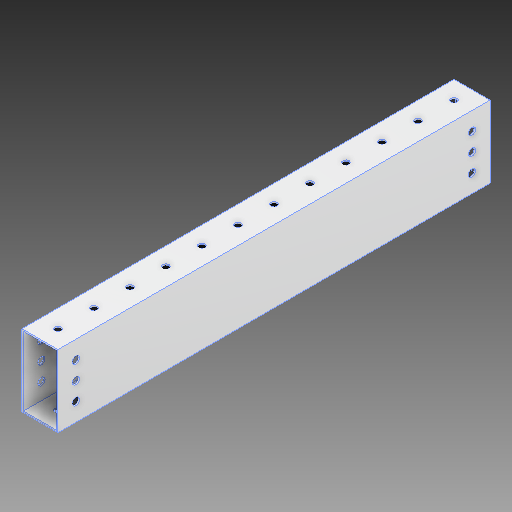
# Autodesk Inventor part: Elevator Stage 1 Gearbox Mounting Tube
Saved by Autodesk Inventor 2022 (Build 260153000, 153)
## iProperties
Created: 2020-09-06
Part Number: Elevator Stage 1 Gearbox Mounting Tube
Material: Aluminum 6061
Document SubType Name: Modeling
Density: 2.7 g/cm^3
Appearance: Aluminum - Flat
Autodesk Inventor part; units mm, degrees
ref_plane "YZ Plane" through (0, 0, 0) normal (1, 0, 0) x (0, 1, 0)
ref_plane "XZ Plane" through (0, 0, 0) normal (0, 1, 0) x (-1, 0, 0)
ref_plane "XY Plane" through (0, 0, 0) normal (0, 0, 1) x (1, 0, 0)
sketch "Sketch1" plane through (0, 0, 0) normal (0, 0, 1) x (1, 0, 0)
  line L0 (12.7, 25.4) -> (-12.7, 25.4)
  line L1 (-12.7, 25.4) -> (-12.7, -25.4)
  line L2 (-12.7, -25.4) -> (12.7, -25.4)
  line L3 (12.7, -25.4) -> (12.7, 25.4)
  line L4 (12.7, 25.4) -> (-12.7, -25.4) construction
  line L5 (-12.7, 25.4) -> (12.7, -25.4) construction
  line L6 (-11.684, 24.384) -> (11.684, 24.384)
  line L7 (11.684, 24.384) -> (11.684, -24.384)
  line L8 (11.684, -24.384) -> (-11.684, -24.384)
  line L9 (-11.684, -24.384) -> (-11.684, 24.384)
  point P0 (0, 0)
  dimension "d0" = 1.016
  dimension "d1" = 50.8
  dimension "d2" = 25.4
  constraints: 20 end point, 4 parallel, 2 midpoint, 2 perpendicular, 1 horizontal, 3 other
  measures "d0" distance between parallel lines of L0 L6
  measures "d1" distance between parallel lines of L2 L0
  measures "d2" distance between parallel lines of L1 L3
extrude "Tube Length" add sketch "Sketch1" along normal mid plane 304.8
sketch "Sketch2" plane through (-12.7, 25.4, 152.4) normal (0, 1, 0) x (1, 0, 0)
  line L0 (0, 0) -> (0, 304.8) projected
  line L1 (25.4, 0) -> (0, 0) projected
  line L2 (25.4, 304.8) -> (25.4, 0) projected
  line L3 (0, 304.8) -> (25.4, 304.8) projected
  line L4 (25.4, 0) -> (0, 0) projected
  line L5 (12.7, 0) -> (12.7, 12.7) construction
  circle A0 centre (12.7, 12.7) radius 2.2479
  point P0 (12.7, 152.4)
  dimension "d5" = 12.7
  dimension "d6" = 4.4958
  constraints: 2 end point, 1 centre point, 1 coincident, 1 midpoint, 1 vertical
  measures "d5" distance of L5.start L5.end
  measures "d6" diameter of A0
extrude "Top Hole" cut sketch "Sketch2" against normal through all contours A0
pattern_linear "Rectangular Pattern1" count 12 spacing 25.4 along (0, 0, -1) of "Top Hole"
sketch "Sketch4" plane through (-12.7, -25.4, 152.4) normal (-1, 0, 0) x (0, 0, 1)
  line L0 (-304.8, 0) -> (0, 0) projected
  line L1 (0, 50.8) -> (0, 0) projected
  line L2 (0, 50.8) -> (-304.8, 50.8) projected
  line L3 (-304.8, 0) -> (-304.8, 50.8) projected
  line L4 (-304.8, 25.4) -> (-292.1, 25.4)
  line L5 (-152.4, 25.4) -> (-152.4, 13.4487)
  point P0 (-292.1, 12.7)
  point P1 (-292.1, 38.1)
  point P2 (-12.7, 12.7)
  point P3 (-12.7, 25.4)
  point P4 (-12.7, 38.1)
  dimension "d31" = 12.7
  dimension "d34" = 12.7
  constraints: 4 end point, 3 symmetric about line, 2 vertical, 1 coincident, 1 horizontal, 1 midpoint, 2 other
  measures "d31" distance of L4.start L4.end
  measures "d34" distance of point (-292.1, 12.7) point (-292.1, 25.4)
hole "Hole1" at (-12.7, -12.7, -139.7) at (-12.7, 0, -139.7) at (-12.7, 12.7, -139.7) at (-12.7, 12.7, 139.7) at (-12.7, -12.7, 139.7) at (-12.7, 0, 139.7) direction (1, 0, 0) diameter 5.1054 end through all clearance for "Flat Head Machine Screw (82)" size "#10" standard "Ansi Unified Screw Threads"
sketch "Sketch3" plane through (0, 0, 152.4) normal (0, 0, 1) x (1, 0, 0)
  line L0 (0, 0) -> (0, 25.4) construction
  line L1 (12.7, 25.4) -> (-12.7, 25.4) projected
  line L2 (-0.0508, 25.4) -> (0, 25.2984)
  line L3 (0.0508, 25.4) -> (0, 25.2984)
  line L4 (-12.7, 12.6492) -> (-12.5984, 12.7)
  line L5 (-12.7, 12.7508) -> (-12.5984, 12.7)
  line L6 (-12.7, -0.0508) -> (-12.5984, 0)
  line L7 (-12.7, 0.0508) -> (-12.5984, 0)
  line L8 (-12.7, -12.7508) -> (-12.5984, -12.7)
  line L9 (-12.7, -12.6492) -> (-12.5984, -12.7)
  line L10 (12.7, 0.0508) -> (12.5984, 0)
  line L11 (12.7, 12.6492) -> (12.5984, 12.7)
  line L12 (12.7, 12.7508) -> (12.5984, 12.7)
  line L13 (12.7, -0.0508) -> (12.5984, 0)
  line L14 (12.7, -12.6492) -> (12.5984, -12.7)
  line L15 (12.7, -12.7508) -> (12.5984, -12.7)
  line L16 (0.0508, -25.4) -> (0, -25.2984)
  line L17 (-0.0508, -25.4) -> (0, -25.2984)
  line L18 (-12.7, 25.4) -> (-12.7, -25.4) projected
  line L19 (12.7, -25.4) -> (12.7, 25.4) projected
  line L20 (-12.7, -25.4) -> (12.7, -25.4) projected
  point P0 (0, 12.7)
  point P1 (-12.7, 12.7)
  point P2 (-12.7, 0)
  point P3 (-12.7, -12.7)
  point P4 (12.7, 12.7)
  point P5 (12.7, 0)
  point P6 (12.7, -12.7)
  point P7 (0, -25.4)
  dimension "d12" = 0.1016
  dimension "d13" = 0.1016
  dimension "d16" = 90
  dimension "d20" = 12.7
  dimension "d27" = 360
  constraints: 34 end point, 3 point on line, 2 midpoint, 2 vertical, 1 equal length, 70 other
  measures "d12" distance of L3.start L2.start
  measures "d13" distance from line of L1 L2.end
  measures "d20" distance of point (-12.7, 12.7) point (-12.7, 0)
equation "\"d13\" = d12"
body "Solid1"
